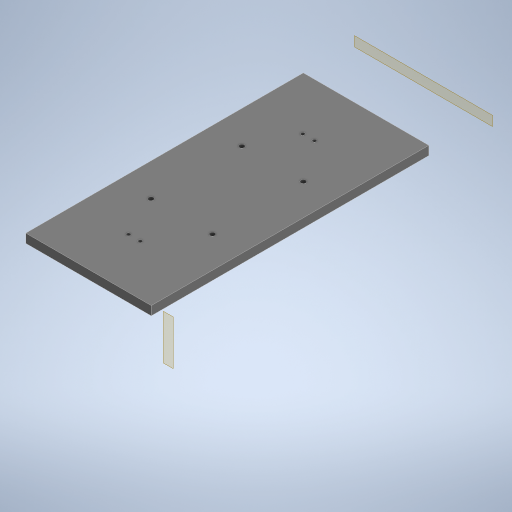
# Autodesk Inventor part: 12_CPY1
Saved by Autodesk Inventor 2024.3 (Build 283343000, 343)
## iProperties
Created: 2024-09-08
Part Number: 12_CPY1
Material: 아크릴, 선명
Document SubType Name: Modeling
Designer: 구지현
Density: 1.19 g/cm^3
Appearance: 회색
Mass: 114.027 g
Surface Area: 353.106 cm^2
Volume: 95.8211 cm^3
Author: 구지현
Autodesk Inventor part; units mm, degrees
ref_plane "YZ Plane" through (0, 0, 0) normal (1, 0, 0) x (0, 1, 0)
ref_plane "XZ Plane" through (0, 0, 0) normal (0, 1, 0) x (-1, 0, 0)
ref_plane "XY Plane" through (0, 0, 0) normal (0, 0, 1) x (1, 0, 0)
ref_plane "작업 평면1" through (-11.501, -90.6951, 25.5) normal (0, 0, 1) x (0, 1, 0)
ref_plane "작업 평면2" through (-154.4039, 73.8066, -132.8958) normal (0, 0, 1) x (0, 1, 0)
sketch "스케치12" plane through (0, 0, 0) normal (0, 1, 0) x (-1, 0, 0)
  line L0 (-42.5, -94) -> (42.5, -94)
  line L1 (42.5, -94) -> (42.5, 94)
  line L2 (42.5, 94) -> (-42.5, 94)
  line L3 (-42.5, 94) -> (-42.5, -94)
  line L4 (-42.5, -94) -> (42.5, 94) construction
  line L5 (42.5, -94) -> (-42.5, 94) construction
  point P0 (0, 0)
  dimension "d71" = 85
  dimension "d72" = 188
  constraints: 12 end point, 2 midpoint, 2 parallel, 1 horizontal, 1 perpendicular
  measures "d71" distance of L2.end L1.end
  measures "d72" distance of L1.end L0.end
extrude "돌출11" add sketch "스케치12" along normal blind 6
sketch "스케치15" plane through (0, 6, 0) normal (0, 1, 0) x (1, 0, 0)
  circle A0 centre (0.9906, -59.9526) radius 1.25 projected
  circle A1 centre (-7.0094, -59.9526) radius 1.25 projected
  line L0 (-13.0094, -54.9526) -> (6.9906, -54.9526) projected
  line L1 (-13.0094, -54.9526) -> (-13.0094, -64.9526) projected
  line L2 (6.9906, -64.9526) -> (-13.0094, -64.9526) projected
  line L3 (6.9906, -54.9526) -> (6.9906, -64.9526) projected
  circle A2 centre (-7.0094, 58.0474) radius 1.25 projected
  circle A3 centre (0.9906, 58.0474) radius 1.25 projected
  line L4 (6.9906, 53.0474) -> (-13.0094, 53.0474) projected
  line L5 (6.9906, 53.0474) -> (6.9906, 63.0474) projected
  line L6 (-13.0094, 63.0474) -> (6.9906, 63.0474) projected
  line L7 (-13.0094, 53.0474) -> (-13.0094, 63.0474) projected
  point P0 (0, 0)
extrude "돌출14" cut sketch "스케치15" against normal blind 10 contours A0 | A1 | A2 | A3
sketch "스케치16" plane through (0, 6, 0) normal (0, 1, 0) x (1, 0, 0)
  circle A0 centre (-20.331, -31.4129) radius 1.6 projected
  circle A1 centre (-20.4117, 30.1871) radius 1.6 projected
  circle A2 centre (21.269, -31.3584) radius 1.6 projected
  circle A3 centre (21.1883, 30.2416) radius 1.6 projected
  line L0 (-24.6171, 34.3816) -> (-24.5254, -35.6184) projected
  line L1 (-24.5254, -35.6184) -> (25.4745, -35.5529) projected
  line L2 (25.4745, -35.5529) -> (25.3828, 34.4471) projected
  line L3 (25.3828, 34.4471) -> (-24.6171, 34.3816) projected
  line L4 (-3.012, -16.0318) -> (-3.013, -15.2211) projected
  line L5 (-3.013, -15.2211) -> (2.3653, -15.2141) projected
  line L6 (2.3653, -15.2141) -> (2.3626, -13.1675) projected
  line L7 (2.3626, -13.1675) -> (3.0843, -13.1666) projected
  line L8 (3.0843, -13.1666) -> (3.0907, -18.0703) projected
  line L9 (3.0907, -18.0703) -> (2.369, -18.0713) projected
  line L10 (2.369, -18.0713) -> (2.3663, -16.0248) projected
  line L11 (2.3663, -16.0248) -> (-3.012, -16.0318) projected
  spline S0 degree 2 poles (-2.5863, -8.9228) (-2.8733, -8.6315) (-3.1512, -7.8607) (-3.1519, -7.2972) knots 0 0 0 1 2 2 2 projected
  spline S1 degree 2 poles (-3.1519, -7.2972) (-3.1526, -6.7584) (-2.8719, -5.9572) (-2.5905, -5.6751) knots 0 0 0 1 2 2 2 projected
  spline S2 degree 2 poles (-2.5905, -5.6751) (-2.2746, -5.3534) (-1.3851, -5.0902) (-0.7326, -5.0893) knots 0 0 0 1 2 2 2 projected
  line L12 (-0.7326, -5.0893) -> (3.0737, -5.0844) projected
  line L13 (3.0737, -5.0844) -> (3.0748, -5.895) projected
  line L14 (3.0748, -5.895) -> (-0.7315, -5.9) projected
  spline S3 degree 2 poles (-0.7315, -5.9) (-1.1567, -5.9006) (-1.7299, -6.0101) (-1.9621, -6.1636) knots 0 0 0 1 2 2 2 projected
  spline S4 degree 2 poles (-1.9621, -6.1636) (-2.209, -6.3271) (-2.4604, -6.891) (-2.4599, -7.2963) knots 0 0 0 1 2 2 2 projected
  spline S5 degree 2 poles (-2.4599, -7.2963) (-2.4594, -7.6769) (-2.2065, -8.2698) (-1.9591, -8.4326) knots 0 0 0 1 2 2 2 projected
  spline S6 degree 2 poles (-1.9591, -8.4326) (-1.7266, -8.5855) (-1.1579, -8.6935) (-0.7477, -8.693) knots 0 0 0 1 2 2 2 projected
  line L15 (-0.7477, -8.693) -> (3.0784, -8.688) projected
  line L16 (3.0784, -8.688) -> (3.0795, -9.4987) projected
  line L17 (3.0795, -9.4987) -> (-0.7268, -9.5037) projected
  spline S7 degree 2 poles (-0.7268, -9.5037) (-1.3645, -9.5045) (-2.2744, -9.2487) (-2.5863, -8.9228) knots 0 0 0 1 2 2 2 projected
  line L18 (-2.4181, 6.0803) -> (-3.0409, 6.0794) projected
  line L19 (-3.0409, 6.0794) -> (-3.044, 8.4423) projected
  line L20 (-3.044, 8.4423) -> (-2.4212, 8.4431) projected
  line L21 (-2.4212, 8.4431) -> (-2.4201, 7.6671) projected
  line L22 (-2.4201, 7.6671) -> (2.4341, 7.6734) projected
  line L23 (2.4341, 7.6734) -> (2.4331, 8.4495) projected
  line L24 (2.4331, 8.4495) -> (3.056, 8.4503) projected
  line L25 (3.056, 8.4503) -> (3.0591, 6.0874) projected
  line L26 (3.0591, 6.0874) -> (2.4362, 6.0866) projected
  line L27 (2.4362, 6.0866) -> (2.4352, 6.8627) projected
  line L28 (2.4352, 6.8627) -> (-2.4191, 6.8564) projected
  line L29 (-2.4191, 6.8564) -> (-2.4181, 6.0803) projected
  spline S8 degree 2 poles (-2.9765, 9.7722) (-3.0659, 10.039) (-3.1555, 10.4936) (-3.1559, 10.8594) knots 0 0 0 1 2 2 2 projected
  spline S9 degree 2 poles (-3.1559, 10.8594) (-3.1567, 11.4526) (-2.7576, 12.4566) (-2.3577, 12.823) knots 0 0 0 1 2 2 2 projected
  spline S10 degree 2 poles (-2.3577, 12.823) (-1.9627, 13.1893) (-0.7769, 13.5913) (-0.0057, 13.5923) knots 0 0 0 1 2 2 2 projected
  spline S11 degree 2 poles (-0.0057, 13.5923) (0.7605, 13.5933) (1.898, 13.2042) (2.3186, 12.834) knots 0 0 0 1 2 2 2 projected
  spline S12 degree 2 poles (2.3186, 12.834) (2.7294, 12.4688) (3.1608, 11.4708) (3.1616, 10.8529) knots 0 0 0 1 2 2 2 projected
  spline S13 degree 2 poles (3.1616, 10.8529) (3.162, 10.5464) (3.0737, 10.0075) (3.0048, 9.78) knots 0 0 0 1 2 2 2 projected
  spline S14 degree 2 poles (3.0048, 9.78) (2.9408, 9.5822) (2.7584, 9.1716) (2.65, 8.9688) knots 0 0 0 1 2 2 2 projected
  line L30 (2.65, 8.9688) -> (1.6712, 8.9675) projected
  line L31 (1.6712, 8.9675) -> (1.6711, 9.0318) projected
  spline S15 degree 2 poles (1.6711, 9.0318) (1.7698, 9.1407) (2.0462, 9.4772) (2.1794, 9.7196) knots 0 0 0 1 2 2 2 projected
  spline S16 degree 2 poles (2.1794, 9.7196) (2.3076, 9.9521) (2.47, 10.501) (2.4695, 10.8569) knots 0 0 0 1 2 2 2 projected
  spline S17 degree 2 poles (2.4695, 10.8569) (2.469, 11.2474) (2.1468, 11.944) (1.84, 12.2056) knots 0 0 0 1 2 2 2 projected
  spline S18 degree 2 poles (1.84, 12.2056) (1.5282, 12.4623) (0.5837, 12.7477) (-0.0046, 12.747) knots 0 0 0 1 2 2 2 projected
  spline S19 degree 2 poles (-0.0046, 12.747) (-0.6324, 12.7461) (-1.5366, 12.4434) (-1.8477, 12.181) knots 0 0 0 1 2 2 2 projected
  spline S20 degree 2 poles (-1.8477, 12.181) (-2.1489, 11.9236) (-2.4545, 11.2361) (-2.454, 10.8505) knots 0 0 0 1 2 2 2 projected
  spline S21 degree 2 poles (-2.454, 10.8505) (-2.4535, 10.4995) (-2.2797, 9.9016) (-2.1509, 9.6694) knots 0 0 0 1 2 2 2 projected
  spline S22 degree 2 poles (-2.1509, 9.6694) (-2.0221, 9.4472) (-1.7547, 9.1163) (-1.6607, 9.0225) knots 0 0 0 1 2 2 2 projected
  line L32 (-1.6607, 9.0225) -> (-1.6606, 8.9632) projected
  line L33 (-1.6606, 8.9632) -> (-2.6295, 8.9619) projected
  spline S23 degree 2 poles (-2.6295, 8.9619) (-2.7236, 9.1645) (-2.8971, 9.5202) (-2.9765, 9.7722) knots 0 0 0 1 2 2 2 projected
  line L34 (-0.3817, 2.5287) -> (-3.0334, 0.3551) projected
  line L35 (-3.0334, 0.3551) -> (-3.0348, 1.4081) projected
  line L36 (-3.0348, 1.4081) -> (-0.6102, 3.3391) projected
  line L37 (-0.6102, 3.3391) -> (-0.6114, 4.2684) projected
  line L38 (-0.6114, 4.2684) -> (-3.0385, 4.2653) projected
  line L39 (-3.0385, 4.2653) -> (-3.0396, 5.076) projected
  line L40 (-3.0396, 5.076) -> (3.0604, 5.084) projected
  line L41 (3.0604, 5.084) -> (3.0625, 3.512) projected
  spline S24 degree 2 poles (3.0625, 3.512) (3.0631, 2.988) (2.9504, 2.281) (2.7432, 1.9594) knots 0 0 0 1 2 2 2 projected
  spline S25 degree 2 poles (2.7432, 1.9594) (2.536, 1.6378) (1.8889, 1.2662) (1.4094, 1.2656) knots 0 0 0 1 2 2 2 projected
  spline S26 degree 2 poles (1.4094, 1.2656) (0.7421, 1.2647) (-0.1635, 1.9457) (-0.3817, 2.5287) knots 0 0 0 1 2 2 2 projected
  spline S27 degree 2 poles (-2.959, -3.5994) (-3.0484, -3.3326) (-3.1379, -2.8779) (-3.1384, -2.5121) knots 0 0 0 1 2 2 2 projected
  spline S28 degree 2 poles (-3.1384, -2.5121) (-3.1392, -1.9189) (-2.7401, -0.9149) (-2.3402, -0.5486) knots 0 0 0 1 2 2 2 projected
  spline S29 degree 2 poles (-2.3402, -0.5486) (-1.9452, -0.1823) (-0.7593, 0.2197) (0.0118, 0.2207) knots 0 0 0 1 2 2 2 projected
  spline S30 degree 2 poles (0.0118, 0.2207) (0.778, 0.2217) (1.9155, -0.1673) (2.3362, -0.5375) knots 0 0 0 1 2 2 2 projected
  spline S31 degree 2 poles (2.3362, -0.5375) (2.7469, -0.9028) (3.1783, -1.9007) (3.1791, -2.5187) knots 0 0 0 1 2 2 2 projected
  spline S32 degree 2 poles (3.1791, -2.5187) (3.1795, -2.8251) (3.0912, -3.3641) (3.0223, -3.5916) knots 0 0 0 1 2 2 2 projected
  spline S33 degree 2 poles (3.0223, -3.5916) (2.9583, -3.7894) (2.776, -4.1999) (2.6675, -4.4027) knots 0 0 0 1 2 2 2 projected
  line L42 (2.6675, -4.4027) -> (1.6887, -4.404) projected
  line L43 (1.6887, -4.404) -> (1.6886, -4.3397) projected
  spline S34 degree 2 poles (1.6886, -4.3397) (1.7873, -4.2309) (2.0637, -3.8943) (2.1969, -3.652) knots 0 0 0 1 2 2 2 projected
  spline S35 degree 2 poles (2.1969, -3.652) (2.3251, -3.4194) (2.4875, -2.8705) (2.487, -2.5146) knots 0 0 0 1 2 2 2 projected
  spline S36 degree 2 poles (2.487, -2.5146) (2.4865, -2.1241) (2.1643, -1.4275) (1.8575, -1.1659) knots 0 0 0 1 2 2 2 projected
  spline S37 degree 2 poles (1.8575, -1.1659) (1.5457, -0.9093) (0.6012, -0.6238) (0.0129, -0.6246) knots 0 0 0 1 2 2 2 projected
  spline S38 degree 2 poles (0.0129, -0.6246) (-0.6149, -0.6254) (-1.5191, -0.9281) (-1.8302, -1.1905) knots 0 0 0 1 2 2 2 projected
  spline S39 degree 2 poles (-1.8302, -1.1905) (-2.1314, -1.448) (-2.437, -2.1355) (-2.4365, -2.5211) knots 0 0 0 1 2 2 2 projected
  spline S40 degree 2 poles (-2.4365, -2.5211) (-2.436, -2.872) (-2.2622, -3.4699) (-2.1334, -3.7021) knots 0 0 0 1 2 2 2 projected
  spline S41 degree 2 poles (-2.1334, -3.7021) (-2.0046, -3.9244) (-1.7372, -4.2552) (-1.6431, -4.349) knots 0 0 0 1 2 2 2 projected
  line L44 (-1.6431, -4.349) -> (-1.6431, -4.4084) projected
  line L45 (-1.6431, -4.4084) -> (-2.6119, -4.4096) projected
  spline S42 degree 2 poles (-2.6119, -4.4096) (-2.7061, -4.2071) (-2.8796, -3.8514) (-2.959, -3.5994) knots 0 0 0 1 2 2 2 projected
  line L46 (-2.3933, -12.7931) -> (-3.0162, -12.794) projected
  line L47 (-3.0162, -12.794) -> (-3.0193, -10.4311) projected
  line L48 (-3.0193, -10.4311) -> (-2.3964, -10.4303) projected
  line L49 (-2.3964, -10.4303) -> (-2.3954, -11.2064) projected
  line L50 (-2.3954, -11.2064) -> (2.4589, -11.2) projected
  line L51 (2.4589, -11.2) -> (2.4579, -10.4239) projected
  line L52 (2.4579, -10.4239) -> (3.0807, -10.4231) projected
  line L53 (3.0807, -10.4231) -> (3.0838, -12.786) projected
  line L54 (3.0838, -12.786) -> (2.4609, -12.7868) projected
  line L55 (2.4609, -12.7868) -> (2.4599, -12.0107) projected
  line L56 (2.4599, -12.0107) -> (-2.3944, -12.017) projected
  line L57 (-2.3944, -12.017) -> (-2.3933, -12.7931) projected
  circle A4 centre (-20.331, -31.4129) radius 1.7
  circle A5 centre (-20.4117, 30.1871) radius 1.7
  circle A6 centre (21.1883, 30.2416) radius 1.7
  circle A7 centre (21.269, -31.3584) radius 1.7
  point P0 (0, 0)
  dimension "d81" = 0.1
  dimension "d82" = 0.1
  dimension "d83" = 0.1
  dimension "d84" = 0.1
  constraints: 4 centre point
  measures "d81" radial gap between concentric circles of A0 A4
  measures "d82" radial gap between concentric circles of A1 A5
  measures "d83" radial gap between concentric circles of A3 A6
  measures "d84" radial gap between concentric circles of A2 A7
extrude "돌출15" cut sketch "스케치16" against normal blind 10 contours A0 | A1 | A2 | A3 | A4 | A5 | A6 | A7
